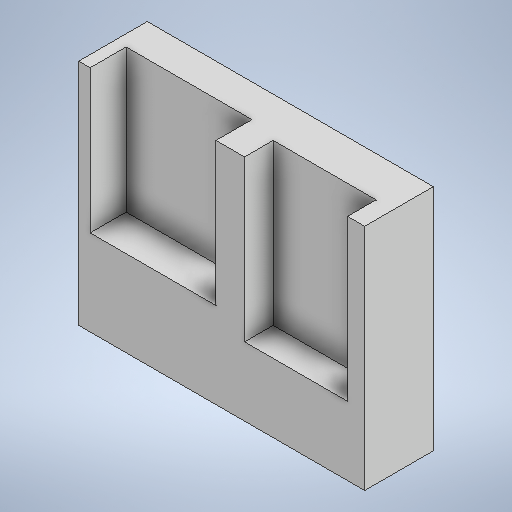
# Autodesk Inventor part: Motorhalterung
Saved by Autodesk Inventor 2025 (Build 290162000, 162)
## iProperties
Created: 2026-06-23
Part Number: Motorhalterung
Material: Generisch
Document SubType Name: Modeling
Designer: GemmiDad-GBSE
Density: 1 g/cm^3
Appearance: Vorgabe
Author: GemmiDad-GBSE
Autodesk Inventor part; units mm, degrees
ref_plane "YZ Plane" through (0, 0, 0) normal (1, 0, 0) x (0, 1, 0)
ref_plane "XZ Plane" through (0, 0, 0) normal (0, 1, 0) x (-1, 0, 0)
sketch "Skizze1" plane through (0, 0, 0) normal (0, 0, 1) x (1, 0, 0)
  line L0 (0, 0) -> (50, 0)
  line L1 (50, 0) -> (50, 12)
  line L2 (50, 12) -> (0, 12)
  line L3 (0, 12) -> (0, 0)
  constraints: 8 end point, 2 parallel, 1 horizontal, 1 perpendicular
extrude "Extrusion1" add sketch "Skizze1" along normal blind 40
ref_plane "Arbeitsebene1" through (0, 0, 40) normal (0, 0, 1) x (1, 0, 0)
sketch "Skizze2" plane through (0, 0, 40) normal (0, 0, 1) x (1, 0, 0)
  line L0 (29, 0) -> (47, 0)
  line L1 (47, 0) -> (47, 5)
  line L2 (47, 5) -> (29, 5)
  line L3 (29, 5) -> (29, 0)
  constraints: 8 end point, 2 parallel, 1 horizontal, 1 perpendicular
extrude "Extrusion2" cut sketch "Skizze2" against normal blind 28
sketch "Skizze3" plane through (0, 0, 40) normal (0, 0, 1) x (1, 0, 0)
  line L0 (2, 0) -> (24, 0)
  line L1 (24, 0) -> (24, 6.3)
  line L2 (24, 6.3) -> (2, 6.3)
  line L3 (2, 6.3) -> (2, 0)
  constraints: 8 end point, 2 parallel, 1 horizontal, 1 perpendicular
extrude "Extrusion3" cut sketch "Skizze3" against normal blind 25
sketch "Skizze4" plane through (0, 0, 0) normal (0, 1, 0) x (-1, 0, 0)
  circle A0 centre (38, 20) radius 2
  constraints: 1 centre point
extrude "Extrusion4" cut sketch "Skizze4" along normal mid plane 30
sketch "Skizze5" plane through (0, 0, 40) normal (0, 0, 1) x (1, 0, 0)
  circle A0 centre (13, 0) radius 2.5
  constraints: 1 centre point
extrude "Extrusion5" cut sketch "Skizze5" against normal blind 5
sketch "Skizze6" plane through (0, 0, 0) normal (0, 0, 1) x (1, 0, 0)
  circle A0 centre (4, -8) radius 2.1
  circle A1 centre (4, 8) radius 2.1
  circle A2 centre (46, -8) radius 2.1
  circle A3 centre (46, 8) radius 2.1
  constraints: 4 centre point
extrude "Extrusion6" cut sketch "Skizze6" along normal blind 5
